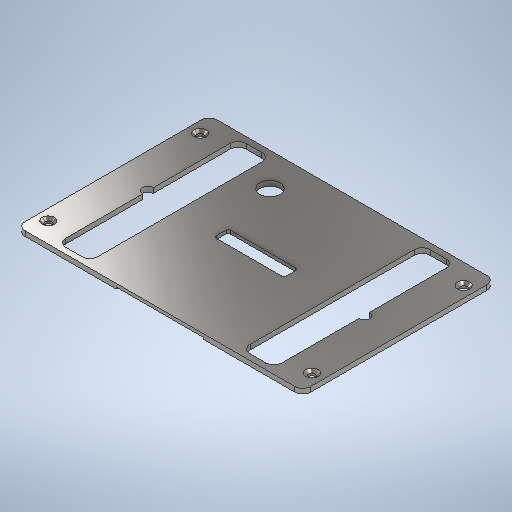
# Autodesk Inventor part: spacer
Saved by Autodesk Inventor 2025 (Build 290162000, 162)
## iProperties
Created: 2021-07-16
Part Number: spacer
Material: Stainless Steel
Document SubType Name: Modeling
Designer: Caleb
Density: 8 g/cm^3
Appearance: Semi-Polished
Author: Caleb
Autodesk Inventor part; units mm, degrees
ref_plane "YZ Plane" through (0, 0, 0) normal (1, 0, 0) x (0, 1, 0)
ref_plane "XZ Plane" through (0, 0, 0) normal (0, 1, 0) x (-1, 0, 0)
ref_plane "XY Plane" through (0, 0, 0) normal (0, 0, 1) x (1, 0, 0)
sketch "Sketch1" plane through (0, 0, 0) normal (0, 1, 0) x (-1, 0, 0)
  line L0 (-35.75, 24.05) -> (35.75, 24.05)
  line L1 (35.75, 24.05) -> (35.75, -24.05)
  line L2 (35.75, -24.05) -> (-35.75, -24.05)
  line L3 (-35.75, -24.05) -> (-35.75, 24.05)
  line L4 (-35.75, 24.05) -> (35.75, -24.05) construction
  line L5 (35.75, 24.05) -> (-35.75, -24.05) construction
  point P0 (0, 0)
  dimension "d0" = 48.1
  dimension "d1" = 71.5
  constraints: 12 end point, 8 point on line, 2 midpoint, 2 parallel, 1 horizontal, 1 perpendicular
  measures "d0" distance of L5.start L4.end
  measures "d1" distance of L4.end L5.end
extrude "Extrusion1" add sketch "Sketch1" along normal blind 1.23
sketch "Sketch2" plane through (0, 1.23, 0) normal (0, 1, 0) x (1, 0, 0)
  point P0 (0, 0)
  point P1 (-33, 19)
  point P2 (33, 19)
  point P3 (-33, -19)
  point P4 (33, -19)
  dimension "d77" = 38
  dimension "d78" = 19
  dimension "d79" = 33
  dimension "d115" = 33
  constraints: 2 horizontal alignment, 2 vertical alignment
  measures "d77" distance of point (-33, -19) point (-33, 19)
  measures "d78" vertical distance of point (-33, 19) point (0, 0)
  measures "d79" horizontal distance of point (-33, 19) point (0, 0)
  measures "d115" horizontal distance of point (0, 0) point (33, 19)
hole "Hole1" at (-33, 1.23, -19) at (33, 1.23, -19) at (-33, 1.23, 19) at (33, 1.23, 19) direction (0, -1, 0) diameter 1.778 end through all countersink diameter 3.023 countersink angle 82 clearance for "Flat Head Machine Screw (82)" size "#0" standard "Ansi Unified Screw Threads"
fillet "Fillet3" radius 2 4 edges at (35.75, 0.615, 24.05) (35.75, 0.615, -24.05) (-35.75, 0.615, -24.05) (-35.75, 0.615, 24.05)
sketch "Sketch10" plane through (0, 1.23, 0) normal (0, 1, 0) x (1, 0, 0)
  line L0 (-27.55, -21) -> (-29.05, -21)
  line L1 (-29.05, -21) -> (-29.05, 21)
  line L2 (-29.05, 21) -> (-27.55, 21)
  line L3 (-27.55, 21) -> (-27.55, -21)
  line L4 (-27.55, -21) -> (-29.05, 21) construction
  line L5 (-29.05, -21) -> (-27.55, 21) construction
  line L6 (0, 13.6561) -> (0, -11.4856)
  line L7 (27.55, -21) -> (29.05, -21)
  line L8 (29.05, -21) -> (29.05, 21)
  line L9 (29.05, 21) -> (27.55, 21)
  line L10 (27.55, 21) -> (27.55, -21)
  line L11 (27.55, -21) -> (29.05, 21) construction
  line L12 (29.05, -21) -> (27.55, 21) construction
  point P0 (0, 0)
  point P1 (-28.3, 0)
  point P2 (-27.55, 0)
  point P3 (28.3, 0)
  point P4 (27.55, 0)
  dimension "d124" = 1.5
  dimension "d125" = 42
  dimension "d126" = 27.55
  constraints: 26 end point, 6 symmetric about line, 3 midpoint, 2 parallel, 1 horizontal, 1 horizontal alignment, 1 perpendicular, 1 point on line, 1 vertical
  measures "d124" distance of L1.end L2.end
  measures "d125" distance of L0.end L1.end
  measures "d126" distance of point (0, 0) point (-27.55, 0)
extrude "Extrusion7" [suppressed]
sketch "Sketch11" plane through (0, 0, 0) normal (0, -1, 0) x (1, 0, 0)
  line L0 (-33.75, 24.05) -> (33.75, 24.05) projected
  line L1 (-11, 24.05) -> (11, 24.05)
  line L2 (11, 24.05) -> (11, -3.95)
  line L3 (9, -5.95) -> (-9, -5.95)
  line L4 (-11, -3.95) -> (-11, 24.05)
  arc A0 (9, -5.95) -> (11, -3.95) centre (9, -3.95) ccw
  arc A1 (-11, -3.95) -> (-9, -5.95) centre (-9, -3.95) ccw
  point P0 (0, 0)
  point P1 (11, -5.95)
  point P2 (-11, -5.95)
  dimension "d129" = 22
  dimension "d130" = 30
  dimension "d131" = 11
  dimension "d132" = 2
  constraints: 8 end point, 5 point on line, 4 point on circle, 4 tangent, 2 centre point, 2 parallel, 1 equal radius, 1 horizontal, 1 perpendicular
  measures "d129" distance of point (11, -5.95) point (-11, -5.95)
  measures "d130" distance of L1.end point (11, -5.95)
  measures "d131" distance from line of L2 point (0, 0)
  measures "d132" radius of A0
extrude "Extrusion8" cut sketch "Sketch11" against normal blind 0.43
sketch "Sketch12" plane through (0, 1.23, 0) normal (0, 1, 0) x (1, 0, 0)
  line L0 (8.25, 1.75) -> (-8.25, 1.75)
  line L1 (-8.75, 1.25) -> (-8.75, -1.25)
  line L2 (-8.25, -1.75) -> (8.25, -1.75)
  line L3 (8.75, -1.25) -> (8.75, 1.25)
  line L4 (8.75, 1.75) -> (-8.75, -1.75) construction
  line L5 (-8.75, 1.75) -> (8.75, -1.75) construction
  arc A0 (-8.75, -1.25) -> (-8.25, -1.75) centre (-8.25, -1.25) ccw
  arc A1 (-8.25, 1.75) -> (-8.75, 1.25) centre (-8.25, 1.25) ccw
  arc A2 (8.25, -1.75) -> (8.75, -1.25) centre (8.25, -1.25) ccw
  arc A3 (8.75, 1.25) -> (8.25, 1.75) centre (8.25, 1.25) ccw
  point P0 (0, 0)
  dimension "d135" = 17.5
  dimension "d136" = 3.5
  dimension "d137" = 0.5
  constraints: 12 end point, 8 point on circle, 8 point on line, 8 tangent, 4 centre point, 3 equal radius, 2 midpoint, 2 parallel, 1 horizontal, 1 perpendicular
  measures "d135" distance of L5.end L4.end
  measures "d136" distance of L5.start L4.end
  measures "d137" radius of A0
extrude "Extrusion9" cut sketch "Sketch12" against normal through all
sketch "Sketch13" plane through (0, 1.23, 0) normal (0, 1, 0) x (1, 0, 0)
  circle A0 centre (-12.25, 15.75) radius 2.5
  point P0 (0, 0)
  dimension "d161" = 15.75
  dimension "d162" = 12.25
  dimension "d163" = 5
  constraints: 1 centre point
  measures "d161" vertical distance of A0.centre point (0, 0)
  measures "d162" horizontal distance of A0.centre point (0, 0)
  measures "d163" diameter of A0
extrude "Extrusion10" cut sketch "Sketch13" against normal through all
sketch "Sketch15" plane through (0, 1.23, 0) normal (0, 1, 0) x (1, 0, 0)
  line L0 (-21.05, -22.55) -> (-25.05, -22.55)
  line L1 (-27.05, -20.55) -> (-27.05, 20.55)
  line L2 (-25.05, 22.55) -> (-21.05, 22.55)
  line L3 (-19.05, 20.55) -> (-19.05, -20.55)
  line L4 (-19.05, -22.55) -> (-27.05, 22.55) construction
  line L5 (-27.05, -22.55) -> (-19.05, 22.55) construction
  arc A0 (-25.05, 22.55) -> (-27.05, 20.55) centre (-25.05, 20.55) ccw
  arc A1 (-27.05, -20.55) -> (-25.05, -22.55) centre (-25.05, -20.55) ccw
  arc A2 (-21.05, -22.55) -> (-19.05, -20.55) centre (-21.05, -20.55) ccw
  arc A3 (-19.05, 20.55) -> (-21.05, 22.55) centre (-21.05, 20.55) ccw
  circle A4 centre (-27.15, 0) radius 1.3
  line L6 (0, 25.2712) -> (0, -27.2079)
  line L7 (21.05, -22.55) -> (25.05, -22.55)
  line L8 (27.05, -20.55) -> (27.05, 20.55)
  line L9 (25.05, 22.55) -> (21.05, 22.55)
  line L10 (19.05, 20.55) -> (19.05, -20.55)
  line L11 (19.05, -22.55) -> (27.05, 22.55) construction
  line L12 (27.05, -22.55) -> (19.05, 22.55) construction
  arc A5 (27.05, 20.55) -> (25.05, 22.55) centre (25.05, 20.55) ccw
  arc A6 (25.05, -22.55) -> (27.05, -20.55) centre (25.05, -20.55) ccw
  arc A7 (19.05, -20.55) -> (21.05, -22.55) centre (21.05, -20.55) ccw
  arc A8 (21.05, 22.55) -> (19.05, 20.55) centre (21.05, 20.55) ccw
  circle A9 centre (27.15, 0) radius 1.3
  point P0 (0, 0)
  point P1 (-23.05, 0)
  point P2 (-27.05, 1.2961)
  point P3 (-27.05, -1.2961)
  point P4 (23.05, 0)
  point P5 (27.05, -1.2961)
  point P6 (27.05, 1.2961)
  dimension "d164" = 45.1
  dimension "d165" = 27.05
  dimension "d166" = 2
  dimension "d167" = 8
  dimension "d170" = 27.15
  dimension "d171" = 2.6
  constraints: 26 end point, 18 symmetric about line, 16 point on circle, 16 point on line, 10 centre point, 8 tangent, 3 equal radius, 2 horizontal alignment, 2 midpoint, 2 parallel, 1 horizontal, 1 perpendicular, 1 vertical, 5 other
  measures "d164" distance of L5.end L4.start
  measures "d165" distance from line of L1 point (0, 0)
  measures "d166" radius of A0
  measures "d167" distance between parallel lines of L1 L3
  measures "d170" distance of A4.centre point (0, 0)
  measures "d171" diameter of A4
extrude "Extrusion11" cut sketch "Sketch15" against normal through all
equation "\"d78\" = 0.5 * d77"
equation "\"d115\" = d79"
equation "\"d131\" = 0.5 * d129"
body "Solid1"
